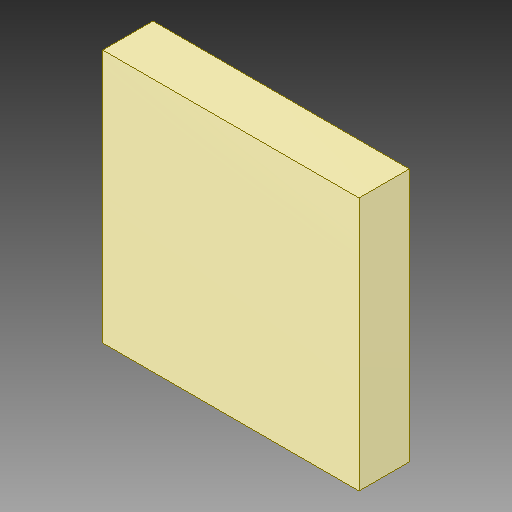
# Autodesk Inventor part: forearm_plate
Saved by Autodesk Inventor 2019 (Build 230136000, 136)
## iProperties
Created: 2024-08-27
Part Number: forearm_plate
Material: Nylon 6/6
Document SubType Name: Modeling
Designer: nic
Density: 1.13 g/cm^3
Appearance: Nylon 6
Author: nic
Autodesk Inventor part; units mm, degrees
ref_plane "YZ Plane" through (0, 0, 0) normal (1, 0, 0) x (0, 1, 0)
ref_plane "XZ Plane" through (0, 0, 0) normal (0, 1, 0) x (-1, 0, 0)
ref_plane "XY Plane" through (0, 0, 0) normal (0, 0, 1) x (1, 0, 0)
sketch "Skizze1" plane through (0, 0, 0) normal (0, 0, 1) x (1, 0, 0)
  line L0 (2.8537, 62.8557) -> (-11.3867, 62.8557) projected
  line L1 (-8.4337, 63.8875) -> (2.8537, 63.8875) projected
  line L2 (2.8537, 63.8875) -> (2.8537, 62.8557) projected
  line L3 (5.1, 52.7557) -> (-5.1, 52.7557)
  line L4 (-5.1, 52.7557) -> (-5.1, 72.9557)
  line L5 (-5.1, 72.9557) -> (5.1, 72.9557)
  line L6 (5.1, 72.9557) -> (5.1, 52.7557)
  line L7 (5.1, 52.7557) -> (-5.1, 72.9557) construction
  line L8 (-5.1, 52.7557) -> (5.1, 72.9557) construction
  line L9 (5.1, 62.8557) -> (-5.1, 62.8557)
  point P0 (0, 0)
  point P1 (0, 62.8557)
  constraints: 14 end point, 4 midpoint, 2 parallel, 1 horizontal, 1 perpendicular, 1 point on line
extrude "Extrusion1" add sketch "Skizze1" along normal blind 2 contours L0 L4 L1 L2 | L2 L1 L4 L5 L6 L9
